Autodesk Inventor part; units mm, degrees
note: some values were not read from the file. Chosen so that the rebuilt part matches the saved one: direction of "Hole2".
(part 15 of 20)
  ellipse E161 centre (8.880264, -22.251224) end of major axis (8.019961, -22.341246) minor radius 0.036963 (9.7365, -22.165406) -> (8.039242, -22.346892) ccw
  ellipse E162 centre (8.776287, -21.257563) end of major axis (9.63659, -21.167541) minor radius 0.036963 (9.63659, -21.167541) -> (8.396683, -21.26386) ccw
  line L202 (9.63659, -21.167541) -> (9.740566, -22.161202)
  line L203 (7.930132, -21.482796) -> (8.019961, -22.341246)
  ellipse E163 centre (-8.87268, -22.249874) end of major axis (-9.732969, -22.159721) minor radius 0.036963 (-8.012398, -22.340088) -> (-9.728903, -22.163926) ccw
  ellipse E164 centre (-8.768552, -21.256229) end of major axis (-9.628841, -21.166076) minor radius 0.036963 (-8.388949, -21.262584) -> (-9.628841, -21.166076) ccw
  line L204 (-7.922432, -21.48159) -> (-8.01239, -22.340027)
  line L205 (-9.628841, -21.166076) -> (-9.732969, -22.159721)
  ellipse E165 centre (7.061717, -21.958191) end of major axis (7.924512, -21.896479) minor radius 0.002538 (7.708444, -21.913617) -> (6.964147, -21.962642) ccw
  line L206 (7.895215, -21.486873) -> (7.924512, -21.896479)
  ellipse E166 centre (9.777958, -21.218746) end of major axis (10.234812, -21.230292) minor radius 0.076505 (9.950925, -21.152163) -> (9.397885, -21.166946) ccw
  ellipse E167 centre (9.777958, -21.218746) end of major axis (10.642682, -21.2406) minor radius 0.144806 (10.484841, -21.319542) -> (9.2764, -21.088429) ccw
  ellipse E168 centre (9.802866, -20.233173) end of major axis (10.66759, -20.255027) minor radius 0.144806 (10.66759, -20.255027) -> (9.58532, -20.087637) ccw
  line L207 (10.66759, -20.255027) -> (10.642682, -21.2406)
  ellipse E169 centre (6.464823, -23.995199) end of major axis (6.018599, -24.093856) minor radius 0.001467 (6.792496, -23.921734) -> (6.030212, -24.091628) ccw
  ellipse E170 centre (6.464823, -23.995199) end of major axis (7.309427, -23.808464) minor radius 0.002777 (6.875465, -23.901925) -> (5.784426, -24.143943) ccw
  ellipse E171 centre (6.248946, -23.018784) end of major axis (7.093549, -22.832049) minor radius 0.002777 (6.975473, -22.856706) -> (5.668507, -23.145047) ccw
  line L208 (9.778285, -23.009543) -> (9.789898, -23.111986)
  line L209 (-9.770816, -23.008056) -> (-9.782444, -23.110498)
  ellipse E172 centre (-6.457505, -23.994216) end of major axis (-6.011296, -24.092941) minor radius 0.001467 (-6.022908, -24.090711) -> (-6.785166, -23.920701) ccw
  ellipse E173 centre (-6.457505, -23.994216) end of major axis (-5.61293, -24.18108) minor radius 0.002777 (-5.926087, -24.109581) -> (-6.868132, -23.90088) ccw
  ellipse E174 centre (-6.241479, -23.017834) end of major axis (-5.396904, -23.204697) minor radius 0.002777 (-5.843014, -23.103486) -> (-6.967981, -22.855645) ccw
  ellipse E175 centre (6.473855, -24.120964) end of major axis (6.919711, -24.020659) minor radius 0.077418 (6.673265, -24.148388) -> (6.070638, -24.174996) ccw
  ellipse E176 centre (6.473855, -24.120964) end of major axis (7.317762, -23.931109) minor radius 0.146534 (6.015845, -24.094803) -> (5.928892, -24.125217) ccw
  ellipse E177 centre (6.473855, -24.120964) end of major axis (7.317762, -23.931109) minor radius 0.146534 (6.927924, -24.148435) -> (7.27682, -23.899258) ccw
  line L210 (7.310373, -23.898267) -> (7.317762, -23.931109)
  ellipse E178 centre (-6.466555, -24.11998) end of major axis (-6.912396, -24.019607) minor radius 0.077418 (-6.057832, -24.177428) -> (-6.579408, -24.172057) ccw
  ellipse E179 centre (-6.466555, -24.11998) end of major axis (-5.622676, -24.309964) minor radius 0.146534 (-5.986709, -24.101247) -> (-6.008541, -24.093889) ccw
  ellipse E180 centre (-6.466555, -24.11998) end of major axis (-7.310434, -23.929997) minor radius 0.146534 (-7.269487, -23.898152) -> (-6.709989, -24.210547) ccw
  line L211 (-7.30304, -23.897155) -> (-7.310434, -23.929997)
  ellipse E181 centre (5.239934, -22.974099) end of major axis (6.04636, -22.661205) minor radius 0.002657 (5.413745, -22.903878) -> (5.065481, -23.039004) ccw
  ellipse E182 centre (4.878209, -22.04182) end of major axis (5.684634, -21.728925) minor radius 0.002657 (5.186609, -21.919528) -> (4.879859, -22.03833) ccw
  ellipse E183 centre (7.817682, -22.838707) end of major axis (8.648839, -22.599117) minor radius 0.158003 (7.952236, -22.639269) -> (7.749399, -22.694025) ccw
  ellipse E184 centre (7.817682, -22.838707) end of major axis (8.648839, -22.599117) minor radius 0.158003 (8.34332, -22.565329) -> (8.005856, -22.626461) ccw
  ellipse E185 centre (-9.875894, -23.012969) end of major axis (-10.332313, -23.03601) minor radius 0.081679 (-9.648403, -22.930955) -> (-9.779917, -23.088231) ccw
  ellipse E186 centre (-9.875894, -23.012969) end of major axis (-10.739794, -23.05658) minor radius 0.1546 (-9.405736, -22.860133) -> (-9.792131, -23.162938) ccw
  ellipse E187 centre (-9.925499, -22.030322) end of major axis (-10.789399, -22.073932) minor radius 0.1546 (-9.702595, -21.86988) -> (-10.789399, -22.073932) ccw
  line L212 (-10.789399, -22.073932) -> (-10.739794, -23.05658)
  ellipse E188 centre (-7.289451, -23.895158) end of major axis (-7.745819, -23.871138) minor radius 0.00147 (-6.894969, -23.916661) -> (-7.061668, -23.908422) ccw
  ellipse E189 centre (-7.289451, -23.895158) end of major axis (-8.153255, -23.849694) minor radius 0.002783 (-6.785011, -23.919446) -> (-7.303056, -23.897228) ccw
  ellipse E190 centre (-7.236891, -22.896545) end of major axis (-6.373087, -22.94201) minor radius 0.002783 (-6.4941, -22.934218) -> (-6.64737, -22.925537) ccw
  ellipse E191 centre (-7.236891, -22.896545) end of major axis (-8.100696, -22.851081) minor radius 0.002783 (-6.734833, -22.920702) -> (-8.100696, -22.851081) ccw
  line L213 (-8.100696, -22.851081) -> (-8.153255, -23.849694)
  ellipse E192 centre (6.236662, -22.702312) end of major axis (5.390447, -22.881603) minor radius 0.130549 (5.390447, -22.881603) -> (7.082877, -22.523021) ccw
  ellipse E193 centre (6.031764, -21.735234) end of major axis (5.185549, -21.914525) minor radius 0.130549 (5.297902, -21.82051) -> (6.83605, -21.610541) ccw
  line L214 (6.888255, -21.604445) -> (7.082877, -22.523021)
  line L215 (5.185549, -21.914525) -> (5.390447, -22.881603)
  ellipse E194 centre (9.046219, -24.203626) end of major axis (9.500344, -24.152445) minor radius 0.009734
  ellipse E195 centre (9.046219, -24.203626) end of major axis (8.18666, -24.300499) minor radius 0.018424 (8.42964, -24.286001) -> (8.202222, -24.302214) ccw
  ellipse E196 centre (8.934252, -23.210142) end of major axis (8.074693, -23.307015) minor radius 0.018424 (9.79381, -23.113269) -> (8.131366, -23.293966) ccw
  line L216 (9.79381, -23.113269) -> (9.905777, -24.106752)
  line L217 (8.136212, -23.852872) -> (8.18666, -24.300499)
  ellipse E197 centre (-9.038932, -24.20225) end of major axis (-9.493049, -24.151001) minor radius 0.009734
  ellipse E198 centre (-9.038932, -24.20225) end of major axis (-9.898475, -24.105246) minor radius 0.018424 (-8.182768, -24.297185) -> (-8.449093, -24.282273) ccw
  ellipse E199 centre (-8.926814, -23.208784) end of major axis (-9.786357, -23.11178) minor radius 0.018424 (-8.123941, -23.29273) -> (-9.786357, -23.11178) ccw
  line L218 (-9.786357, -23.11178) -> (-9.898475, -24.105246)
  ellipse E200 centre (-6.229147, -22.701364) end of major axis (-7.075334, -22.521944) minor radius 0.130549 (-7.075334, -22.521944) -> (-5.382959, -22.880783) ccw
  ellipse E201 centre (-6.024101, -21.734318) end of major axis (-6.870289, -21.554898) minor radius 0.130549 (-6.828368, -21.609501) -> (-5.209084, -21.866915) ccw
  line L219 (-5.177914, -21.913737) -> (-5.382959, -22.880783)
  line L220 (-6.880573, -21.603398) -> (-7.075334, -22.521944)
  ellipse E202 centre (7.296785, -23.896267) end of major axis (6.840413, -23.920218) minor radius 0.00147 (7.068999, -23.909497) -> (6.9023, -23.91771) ccw
  ellipse E203 centre (7.296785, -23.896267) end of major axis (8.160596, -23.850934) minor radius 0.002783 (7.31039, -23.898339) -> (6.792341, -23.920478) ccw
  ellipse E204 centre (7.244377, -22.897647) end of major axis (8.108188, -22.852314) minor radius 0.002783 (6.654851, -22.926548) -> (6.50158, -22.935206) ccw
  ellipse E205 centre (7.244377, -22.897647) end of major axis (8.108188, -22.852314) minor radius 0.002783 (8.108188, -22.852314) -> (6.742315, -22.921727) ccw
  line L221 (8.108188, -22.852314) -> (8.160596, -23.850934)
  ellipse E206 centre (9.883362, -23.014472) end of major axis (10.339777, -23.037582) minor radius 0.081679 (9.787373, -23.089719) -> (9.655883, -22.932423) ccw
  ellipse E207 centre (9.883362, -23.014472) end of major axis (10.747255, -23.058214) minor radius 0.1546 (9.799576, -23.164428) -> (9.413227, -22.861565) ccw
  ellipse E208 centre (9.933116, -22.031832) end of major axis (10.797009, -22.075574) minor radius 0.1546 (10.797009, -22.075574) -> (9.710237, -21.871357) ccw
  line L222 (10.797009, -22.075574) -> (10.747255, -23.058214)
  ellipse E209 centre (-7.810188, -22.837519) end of major axis (-6.979067, -23.077235) minor radius 0.158003 (-7.741883, -22.692847) -> (-7.816372, -22.671587) ccw
  ellipse E210 centre (-5.23246, -22.973303) end of major axis (-4.426082, -23.28632) minor radius 0.002657 (-5.102543, -23.020921) -> (-5.235934, -22.969105) ccw
  ellipse E211 centre (-4.870593, -22.041078) end of major axis (-4.064215, -22.354095) minor radius 0.002657 (-4.916775, -22.020307) -> (-5.105229, -21.947273) ccw
  ellipse E212 centre (8.55857, -18.364881) end of major axis (9.419561, -18.281692) minor radius 0.221488 (9.139361, -18.148216) -> (9.043274, -18.137267) ccw
  ellipse E213 centre (-8.550395, -18.36358) end of major axis (-7.689418, -18.4469) minor radius 0.221488 (-9.035064, -18.135893) -> (-9.131153, -18.146827) ccw
  ellipse E214 centre (-9.638197, -19.369972) end of major axis (-9.181207, -19.366996) minor radius 0.071862 (-9.5006, -19.300569) -> (-9.830873, -19.306032) ccw
  ellipse E215 centre (-9.638197, -19.369972) end of major axis (-10.503179, -19.375606) minor radius 0.13602 (-9.494183, -19.234934) -> (-10.501861, -19.36795) ccw
  ellipse E216 centre (-9.644629, -18.382434) end of major axis (-10.509611, -18.388068) minor radius 0.13602 (-9.049152, -18.279994) -> (-10.504657, -18.37336) ccw
  ellipse E217 centre (8.735192, -20.282112) end of major axis (9.19003, -20.237714) minor radius 0.026267 (9.1877, -20.24076) -> (9.187114, -20.235158) ccw
  ellipse E218 centre (8.735192, -20.282112) end of major axis (9.5961, -20.198076) minor radius 0.049718 (9.586329, -20.206816) -> (8.550212, -20.251321) ccw
  ellipse E219 centre (8.638201, -19.288488) end of major axis (9.499109, -19.204451) minor radius 0.049718 (9.499109, -19.204451) -> (8.704737, -19.23221) ccw
  line L223 (9.499109, -19.204451) -> (9.5961, -20.198076)
  ellipse E220 centre (-8.727309, -20.280784) end of major axis (-9.18214, -20.236316) minor radius 0.026267 (-9.179223, -20.233761) -> (-9.17981, -20.239364) ccw
  ellipse E221 centre (-8.727309, -20.280784) end of major axis (-9.588204, -20.196617) minor radius 0.049718 (-8.542324, -20.250021) -> (-9.578434, -20.205359) ccw
  ellipse E222 centre (-8.630166, -19.287175) end of major axis (-9.491062, -19.203007) minor radius 0.049718 (-8.696694, -19.230887) -> (-9.491062, -19.203007) ccw
  line L224 (-9.491062, -19.203007) -> (-9.588204, -20.196617)
  ellipse E223 centre (9.646219, -19.371439) end of major axis (10.103209, -19.374485) minor radius 0.071862 (9.838905, -19.307528) -> (9.508633, -19.302015) ccw
  ellipse E224 centre (9.646219, -19.371439) end of major axis (10.5112, -19.377204) minor radius 0.13602 (10.509883, -19.369548) -> (9.502226, -19.236378) ccw
  ellipse E225 centre (9.652802, -18.383902) end of major axis (10.517782, -18.389667) minor radius 0.13602 (10.512831, -18.374958) -> (9.05734, -18.281371) ccw
  ellipse E226 centre (0.009553, 53.506137) end of major axis (0.075525, 54.246444) minor radius 0.194882 (0.21457, 53.727796) -> (-0.195464, 53.284479) ccw
  line L225 (-0.195616, 51.274821) -> (-0.195464, 53.284479)
  line L226 (0.214417, 51.717553) -> (0.21457, 53.727796)
  ellipse E227 centre (2.143874, 53.506396) end of major axis (2.287088, 54.260493) minor radius 0.195462 (2.370981, 53.706836) -> (2.096124, 54.036091) ccw
  line L227 (-0.341173, 31.740705) -> (-0.256979, 32.544836)
  line L228 (2.209519, 52.164737) -> (2.370981, 53.706836)
  ellipse E228 centre (-2.124767, 53.50672) end of major axis (-2.140806, 54.274124) minor radius 0.195482 (-2.098936, 54.257488) -> (-2.305492, 53.26384) ccw
  line L229 (-2.200438, 52.259018) -> (-2.305492, 53.26384)
  line L230 (0.356969, 31.740652) -> (0.272897, 32.544796)
  ellipse E229 centre (0.0094, 51.496187) end of major axis (0.075622, 52.233172) minor radius 0.194809 (0.214417, 51.717553) -> (-0.195616, 51.274821) ccw
  line L231 (-0.196874, 34.739571) -> (-0.195616, 51.274821)
  line L232 (0.213126, 34.73954) -> (0.214417, 51.717553)
  ellipse E230 centre (2.174873, 51.495886) end of major axis (2.327161, 52.248199) minor radius 0.195466 (2.404376, 51.693529) -> (2.105864, 51.960619) ccw
  line L233 (-1.161209, 24.726698) -> (-0.341156, 31.740871)
  line L234 (0.224889, 33.051688) -> (2.404376, 51.693529)
  line L235 (-0.197636, 24.724772) -> (-0.197141, 31.229224)
  line L236 (0.212364, 24.724741) -> (0.212859, 31.229193)
  ellipse E231 centre (-2.156072, 51.496216) end of major axis (-2.181353, 52.263368) minor radius 0.195478 (-2.116003, 52.223205) -> (-2.333848, 51.251129) ccw
  line L237 (-0.208894, 33.051721) -> (-2.333848, 51.251129)
  line L238 (1.175938, 24.72652) -> (0.356952, 31.740818)
  ellipse E232 centre (0.009707, 55.534244) end of major axis (0.073644, 56.299137) minor radius 0.195472 (0.214724, 55.757114) -> (-0.195309, 55.311374) ccw
  line L239 (-0.195311, 55.290346) -> (-0.195309, 55.311374)
  line L240 (0.214723, 55.734095) -> (0.214724, 55.757114)
  ellipse E233 centre (0.009706, 55.51222) end of major axis (0.075476, 56.255172) minor radius 0.19494 (0.214723, 55.734095) -> (-0.195311, 55.290346) ccw
  line L241 (-0.195464, 53.284479) -> (-0.195311, 55.290346)
  line L242 (0.21457, 53.727796) -> (0.214723, 55.734095)
  ellipse E234 centre (2.127756, 55.512884) end of major axis (2.2636, 56.268331) minor radius 0.195467 (2.352894, 55.715465) -> (1.902618, 55.310302) ccw
  ellipse E235 centre (-0.793704, 24.716213) end of major axis (-0.58962, 24.696853) minor radius 0.000002 (-0.58962, 24.696853) -> (-0.835491, 24.720179) ccw
  line L243 (-0.257064, 32.543938) -> (-0.208885, 33.051813)
  line L244 (0.213336, 37.502674) -> (1.902618, 55.310302)
  line L245 (-0.58962, 24.696853) -> (-0.197323, 28.832262)
  line L246 (2.211634, 54.22637) -> (2.352894, 55.715465)
  ellipse E236 centre (-2.108345, 55.513206) end of major axis (-2.116886, 56.280719) minor radius 0.195476 (-1.925268, 55.754376) -> (-2.291421, 55.272036) ccw
  ellipse E237 centre (0.808431, 24.716091) end of major axis (0.604345, 24.696762) minor radius 0.000002 (0.850219, 24.720051) -> (0.604345, 24.696762) ccw
  line L247 (0.604345, 24.696762) -> (0.212677, 28.832231)
  line L248 (-2.193994, 54.243342) -> (-2.291421, 55.272036)
  line L249 (0.272982, 32.543898) -> (0.224881, 33.05178)
  line L250 (-0.196664, 37.502705) -> (-1.925268, 55.754376)
  line L251 (-9.047868, -18.018858) -> (-9.022159, -18.0039)
  line L252 (-9.106303, -17.898872) -> (-9.099175, -17.900444)
  line L253 (-9.132668, -17.914212) -> (-9.106303, -17.898872)
  line L254 (-9.106303, -17.898872) -> (-9.103206, -17.868962)
  line L255 (-10.711204, -17.866226) -> (-10.693895, -17.867036)
  line L256 (-10.693895, -17.867036) -> (-10.646494, -17.847198)
  line L257 (-10.542988, -17.803879) -> (-10.509871, -17.790019)
  line L258 (-10.338718, -17.71839) -> (-10.314571, -17.708284)
  line L259 (-10.507779, -17.699245) -> (-10.314571, -17.708284)
  line L260 (-10.589465, -17.733432) -> (-10.507779, -17.699245)
  line L261 (-10.314571, -17.708284) -> (-10.314603, -17.707039)
  line L262 (-10.507779, -17.699245) -> (-10.509198, -17.642731)
  line L263 (-10.555517, -15.798913) -> (-10.555525, -15.79856)
  line L264 (-10.608119, -13.704923) -> (-10.608743, -13.680109)
  line L265 (-9.94401, -17.647378) -> (-9.981118, -17.662908)
  line L266 (-9.944338, -17.634328) -> (-9.94401, -17.647378)
  line L267 (-9.94401, -17.647378) -> (-9.82656, -17.652873)
  line L268 (-9.676661, -17.659886) -> (-9.19249, -17.682536)
  line L269 (9.239478, -17.73124) -> (9.266389, -17.728982)
  line L270 (9.509904, -17.708556) -> (9.518634, -17.707823)
  line L271 (9.773763, -17.64453) -> (9.799149, -17.651722)
  line L272 (9.714512, -17.6495) -> (9.773763, -17.64453)
  line L273 (9.773763, -17.64453) -> (9.774235, -17.625861)
  line L274 (10.194358, -17.601742) -> (10.191995, -17.695228)
  line L275 (10.368223, -17.680446) -> (10.191995, -17.695228)
  line L276 (10.469835, -13.659859) -> (10.469373, -13.678124)
  line L277 (10.416258, -15.779768) -> (10.415723, -15.800971)
  line L278 (10.369921, -17.613254) -> (10.368223, -17.680446)
  line L279 (10.191995, -17.695228) -> (10.315866, -17.730322)
  line L280 (10.598304, -17.810338) -> (10.611283, -17.814015)
  line L281 (10.368223, -17.680446) -> (10.526706, -17.725345)
  line L282 (10.67671, -17.900341) -> (10.658231, -17.895106)
  line L283 (9.134915, -17.754095) -> (9.147769, -17.756408)
  line L284 (-10.64598, -17.972818) -> (-10.871518, -17.96517)
  line L285 (-10.959481, -18.003583) -> (-10.871518, -17.96517)
  line L286 (-10.643886, -18.014285) -> (-10.959481, -18.003583)
  line L287 (-10.959481, -18.003583) -> (-10.961848, -17.956702)
  line L288 (-11.169241, -17.911708) -> (-10.978836, -17.918164)
  line L289 (-11.172014, -17.856777) -> (-11.169241, -17.911708)
  line L290 (-10.978836, -17.918164) -> (-10.572528, -17.740733)
  line L291 (-10.762932, -17.734276) -> (-10.572528, -17.740733)
  line L292 (-11.169241, -17.911708) -> (-10.762932, -17.734276)
  line L293 (-10.572528, -17.740733) -> (-10.572852, -17.734313)
  line L294 (-10.762932, -17.734276) -> (-10.763409, -17.724824)
  line L295 (-10.395036, -13.665397) -> (-10.393502, -13.695801)
  line L296 (9.924361, -17.718581) -> (9.927437, -17.718404)
  line L297 (10.142861, -17.706037) -> (10.201617, -17.702664)
  line L298 (10.094508, -17.665104) -> (10.201617, -17.702664)
  line L299 (10.038776, -17.668304) -> (10.094508, -17.665104)
  line L300 (10.201617, -17.702664) -> (10.201852, -17.698021)
  line L301 (10.094508, -17.665104) -> (10.097435, -17.607306)
  line L302 (10.189858, -15.781958) -> (10.190459, -15.770084)
  line L303 (10.502946, -17.727127) -> (10.502742, -17.731166)
  line L304 (10.683071, -17.720814) -> (10.502742, -17.731166)
  line L305 (10.684038, -17.701713) -> (10.683071, -17.720814)
  line L306 (10.502742, -17.731166) -> (10.99748, -17.904656)
  line L307 (11.17781, -17.894303) -> (10.99748, -17.904656)
  line L308 (10.683071, -17.720814) -> (11.17781, -17.894303)
  line L309 (11.17781, -17.894303) -> (11.180482, -17.841516)
  line L310 (11.027881, -17.992409) -> (10.920773, -17.954849)
  line L311 (11.03036, -17.943446) -> (11.027881, -17.992409)
  line L312 (10.920773, -17.954849) -> (10.654432, -17.97014)
  line L313 (11.027881, -17.992409) -> (10.652212, -18.013976)
  line L314 (-10.130994, -17.702463) -> (-10.064078, -17.680853)
  line L315 (-10.25215, -17.667357) -> (-10.064078, -17.680853)
  line L316 (-10.359884, -17.702149) -> (-10.25215, -17.667357)
  line L317 (-10.064078, -17.680853) -> (-10.064408, -17.630256)
  line L318 (-10.076474, -15.77766) -> (-10.079226, -15.355191)
  line L319 (-10.25215, -17.667357) -> (-10.252433, -17.623881)
  line L320 (-10.264515, -15.768863) -> (-10.264554, -15.76289)
  line L321 (-10.278215, -13.665506) -> (-10.278389, -13.638755)
  line L322 (9.002945, -17.724125) -> (9.727913, -17.663671)
  line L323 (9.623702, -17.634324) -> (9.727913, -17.663671)
  line L324 (9.34766, -17.657343) -> (9.623702, -17.634324)
  line L325 (9.727913, -17.663671) -> (9.727979, -17.653778)
  line L326 (9.623702, -17.634324) -> (9.62385, -17.612121)
  line L327 (9.650348, -13.636669) -> (9.650555, -13.605672)
  line L328 (-7.427478, 0.491287) -> (-8.422703, 0.595367)
  line L329 (-11.2211, 1.390746) -> (-8.370636, 1.092648)
  ellipse E238 centre (-9.068011, 1.165222) end of major axis (-11.554419, 1.425556) minor radius 0.000177 (-11.2211, 1.390746) -> (-11.554419, 1.425556) ccw
  line L330 (-11.752095, -0.462417) -> (-11.554419, 1.425556)
  line L331 (8.433761, 0.594085) -> (7.43852, 0.490157)
  line L332 (8.38177, 1.091374) -> (11.23228, 1.389038)
  ellipse E239 centre (9.079156, 1.163842) end of major axis (11.565604, 1.423798) minor radius 0.000177 (11.565604, 1.423798) -> (11.23228, 1.389038) ccw
  line L333 (11.565604, 1.423798) -> (11.762993, -0.464205)
  ellipse E240 centre (-8.794361, -3.325086) end of major axis (-9.04267, -3.296056) minor radius 0.000013
  ellipse E241 centre (-7.725925, -3.450033) end of major axis (-8.318787, -3.380719) minor radius 0.00003 (-8.267942, -3.386651) -> (-8.267945, -3.386675) ccw
  ellipse E242 centre (-11.214903, -3.042309) end of major axis (-10.424441, -3.134724) minor radius 0.000039 (-11.564379, -3.001416) -> (-11.564487, -3.001473) ccw
  line L334 (-8.26792, -3.386459) -> (-12.108041, -2.937836)
  ellipse E243 centre (-9.957751, -3.189298) end of major axis (-12.440838, -2.898991) minor radius 0.000126 (-12.100681, -2.938696) -> (-12.440795, -2.898995) ccw
  line L335 (-11.817734, -0.454749) -> (-8.971383, -0.787274)
  ellipse E244 centre (-9.667444, -0.706211) end of major axis (-12.150531, -0.415904) minor radius 0.000126 (-11.817734, -0.454749) -> (-12.150531, -0.415904) ccw
  line L336 (-12.440838, -2.898991) -> (-12.150531, -0.415904)
  ellipse E245 centre (-4.295954, -3.851144) end of major axis (-12.73845, -2.864101) minor radius 0.000429 (-12.316833, -2.913529) -> (-11.564641, -3.001555) ccw
  line L337 (-8.035802, -1.399974) -> (-9.029444, -1.283892)
  ellipse E246 centre (8.804824, -3.326425) end of major axis (8.55651, -3.355418) minor radius 0.000013
  ellipse E247 centre (7.736368, -3.451209) end of major axis (8.329241, -3.381985) minor radius 0.00003 (8.278398, -3.387934) -> (8.278395, -3.387909) ccw
  ellipse E248 centre (4.306337, -3.851799) end of major axis (12.748983, -2.866039) minor radius 0.000429 (11.575153, -3.003315) -> (12.327357, -2.915403) ccw
  ellipse E249 centre (9.968234, -3.190813) end of major axis (12.451365, -2.900884) minor radius 0.000126 (12.327357, -2.915403) -> (12.118562, -2.939678) ccw
  line L338 (12.118562, -2.939678) -> (8.278373, -3.387717)
  line L339 (8.982231, -0.78864) -> (11.828633, -0.456547)
  ellipse E250 centre (9.678304, -0.707682) end of major axis (12.161436, -0.417753) minor radius 0.000126 (12.161436, -0.417753) -> (11.828633, -0.456547) ccw
  line L340 (12.161436, -0.417753) -> (12.451365, -2.900884)
  ellipse E251 centre (11.225408, -3.044015) end of major axis (10.434932, -3.13631) minor radius 0.000039 (11.574998, -3.003233) -> (11.574891, -3.003175) ccw
  line L341 (9.040217, -1.285266) -> (8.046557, -1.401197)
  line L342 (-6.927395, 2.406749) -> (-7.923221, 2.501197)
  line L343 (-10.728785, 3.269529) -> (-7.876002, 2.998962)
  ellipse E252 centre (-8.573487, 3.065058) end of major axis (-11.062314, 3.301155) minor radius 0.000028 (-10.728785, 3.269529) -> (-11.062314, 3.301155) ccw
  line L344 (-11.24332, 1.39307) -> (-11.062314, 3.301155)
  line L345 (4.093757, 2.586746) -> (4.005682, 2.601143)
  line L346 (-3.994318, 2.601751) -> (-4.082396, 2.587368)
  line L347 (-5.778862, 2.808104) -> (-4.994293, 2.936222)
  line L348 (5.005707, 2.935462) -> (5.790257, 2.807224)
  line L349 (7.93457, 2.499991) -> (6.938729, 2.405694)
  line L350 (7.887426, 2.997763) -> (10.74025, 3.267897)
  ellipse E253 centre (8.584922, 3.063753) end of major axis (11.073784, 3.299472) minor radius 0.000028 (11.073784, 3.299472) -> (10.74028, 3.267899) ccw
  line L351 (11.073784, 3.299472) -> (11.2545, 1.391359)
  spline S0 degree 3 poles (-6.270261, 3.386408) (-6.22537, 3.406214) (-6.136517, 3.445415) (-6.003702, 3.501576) (-5.872921, 3.555061) (-5.702594, 3.621964) (-5.493969, 3.699586) (-5.32639, 3.754652) (-5.244083, 3.781698) knots 0 0 0 0 0.13378969 0.26480564 0.39318317 0.51905417 0.76378306 1 1 1 1
  line L352 (-6.325383, 2.859948) -> (-6.270261, 3.386408)
  spline S1 degree 3 poles (-7.39801, 3.74416) (-7.41143, 3.74308) (-7.437886, 3.74095) (-7.477008, 3.738874) (-7.514824, 3.737738) (-7.551134, 3.737655) (-7.585748, 3.738663) (-7.618528, 3.740793) (-7.649392, 3.743982) (-7.678296, 3.74818) (-7.705199, 3.753335) (-7.730058, 3.759394) (-7.752833, 3.766308) (-7.773504, 3.774031) (-7.792228, 3.782612) (-7.809155, 3.79217) (-7.824593, 3.802616) (-7.833739, 3.810627) (-7.838227, 3.814557) knots 0 0 0 0 0.08847523 0.17442408 0.25743028 0.33708941 0.41301484 0.48496567 0.5529194 0.61687848 0.67685349 0.73286663 0.78495643 0.83318442 0.87777974 0.92016243 0.96082909 1 1 1 1
  ellipse E254 centre (-3.138193, 3.058154) end of major axis (-8.569503, 3.626827) minor radius 0.000387 (-6.270263, 3.386408) -> (-8.569503, 3.626827) ccw
  line L353 (-8.255694, 3.881151) -> (-8.569503, 3.626827)
  line L354 (-8.627777, 3.070263) -> (-8.569503, 3.626827)
  spline S2 degree 3 poles (-3.144169, 3.522717) (-3.101581, 3.546955) (-3.017287, 3.594929) (-2.891037, 3.664227) (-2.766531, 3.730668) (-2.604086, 3.814476) (-2.404663, 3.912851) (-2.243738, 3.984658) (-2.164694, 4.019928) knots 0 0 0 0 0.13376268 0.26475964 0.39312605 0.51899363 0.76373828 1 1 1 1
  line L355 (-3.144182, 3.340991) -> (-3.144169, 3.522717)
  line L356 (3.155673, 3.522238) -> (3.155659, 3.340512)
  spline S3 degree 3 poles (2.176274, 4.019598) (2.255312, 3.984316) (2.416226, 3.912485) (2.615634, 3.814079) (2.778066, 3.730246) (2.902563, 3.663786) (3.028802, 3.594469) (3.113089, 3.546482) (3.155673, 3.522238) knots 0 0 0 0 0.23626172 0.48100637 0.60687395 0.73524036 0.86623732 1 1 1 1
  line L357 (-2.164694, 4.019928) -> (2.176274, 4.019598)
  ellipse E255 centre (0.005755, 3.555498) end of major axis (-4.955245, 3.555876) minor radius 0.5163 (2.68037, 3.990137) -> (2.176274, 4.019598) ccw
  ellipse E256 centre (0.005755, 3.555498) end of major axis (-4.955245, 3.555876) minor radius 0.5163 (-2.164694, 4.019928) -> (-2.668795, 3.990544) ccw
  ellipse E257 centre (0.005717, 3.058213) end of major axis (5.466717, 3.057798) minor radius 0.568336 (5.303063, 3.195907) -> (3.155673, 3.522238) ccw
  ellipse E258 centre (0.005717, 3.058213) end of major axis (-5.455283, 3.058629) minor radius 0.568336 (-3.144169, 3.522717) -> (-5.291609, 3.196713) ccw
  line L358 (6.281745, 3.385454) -> (6.336786, 2.858985)
  spline S4 degree 3 poles (5.255626, 3.780899) (5.337929, 3.753841) (5.5055, 3.698749) (5.714113, 3.621096) (5.884429, 3.554167) (6.015203, 3.500662) (6.148009, 3.44448) (6.236856, 3.405266) (6.281745, 3.385454) knots 0 0 0 0 0.23621694 0.48094583 0.60681683 0.73519436 0.86621031 1 1 1 1
  spline S5 degree 3 poles (7.849327, 3.813558) (7.844658, 3.809554) (7.835089, 3.801347) (7.818862, 3.790633) (7.800944, 3.780749) (7.781217, 3.771856) (7.759735, 3.763923) (7.736504, 3.756977) (7.711541, 3.751027) (7.684861, 3.746091) (7.656461, 3.74218) (7.626293, 3.739311) (7.594323, 3.737468) (7.56055, 3.736632) (7.525029, 3.736795) (7.487824, 3.737963) (7.448989, 3.740063) (7.422599, 3.742214) (7.409134, 3.743311) knots 0 0 0 0 0.04039145 0.08278851 0.12750015 0.17478558 0.22486002 0.27790108 0.33405492 0.39344169 0.45616024 0.52241148 0.59256068 0.66658365 0.74441779 0.82598879 0.91121312 1 1 1 1
  ellipse E259 centre (3.149626, 3.057676) end of major axis (8.581023, 3.625523) minor radius 0.000387 (8.581023, 3.625523) -> (6.281745, 3.385454) ccw
  line L359 (8.267252, 3.879894) -> (8.581023, 3.625523)
  line L360 (8.639212, 3.06895) -> (8.581023, 3.625523)
  spline S6 degree 3 poles (-5.798085, 5.31307) (-5.753389, 5.333312) (-5.664922, 5.373376) (-5.532661, 5.430829) (-5.402406, 5.485586) (-5.23274, 5.554145) (-5.024881, 5.633795) (-4.857846, 5.690492) (-4.775807, 5.718338) knots 0 0 0 0 0.13378969 0.26480564 0.39318317 0.51905417 0.76378306 1 1 1 1
  line L361 (-5.968571, 3.515891) -> (-5.798085, 5.31307)
  line L362 (-4.775807, 5.718338) -> (-3.980079, 5.642853)
  ellipse E260 centre (-2.615343, 5.51334) end of major axis (-7.554171, 5.981852) minor radius 0.000055 (-7.384376, 5.965759) -> (-7.554171, 5.981852) ccw
  ellipse E261 centre (-2.615343, 5.51334) end of major axis (-7.554171, 5.981852) minor radius 0.000055 (-4.775806, 5.718338) -> (-6.11123, 5.845009) ccw
  spline S7 degree 3 poles (-6.11123, 5.845009) (-6.1628, 5.829169) (-6.263815, 5.798141) (-6.413188, 5.757283) (-6.556182, 5.722285) (-6.691956, 5.693824) (-6.820794, 5.671951) (-6.942412, 5.657483) (-7.038947, 5.651776) (-7.110576, 5.652136) (-7.158813, 5.654891) (-7.202884, 5.659959) (-7.242634, 5.667172) (-7.277945, 5.676377) (-7.317413, 5.690502) (-7.358752, 5.713338) (-7.395931, 5.751237) (-7.416895, 5.798571) (-7.419451, 5.852124) (-7.408266, 5.909059) (-7.39259, 5.946264) (-7.384375, 5.965759) knots 0 0 0 0 0.10413454 0.20397599 0.29888876 0.38827472 0.47171081 0.55106733 0.62459732 0.65820388 0.68929134 0.71781594 0.74378428 0.76721832 0.78816557 0.82463321 0.85738378 0.88888098 0.92222056 0.95924484 1 1 1 1
  ellipse E262 centre (-2.662562, 5.015575) end of major axis (-8.099155, 5.531306) minor radius 0.000061 (-5.798127, 5.313074) -> (-8.099155, 5.531306) ccw
  line L363 (-7.554171, 5.981852) -> (-8.099155, 5.531306)
  ellipse E263 centre (-6.053301, 5.839497) end of major axis (-4.548756, 5.696772) minor radius 0.000017 (-7.384833, 5.965802) -> (-6.193955, 5.852823) ccw
  line L364 (-8.255694, 3.881151) -> (-8.099155, 5.531306)
  spline S8 degree 3 poles (-3.144023, 5.436372) (-3.101436, 5.460633) (-3.017142, 5.508654) (-2.890892, 5.578019) (-2.766386, 5.644525) (-2.603942, 5.728415) (-2.40452, 5.826886) (-2.243592, 5.898764) (-2.164548, 5.934068) knots 0 0 0 0 0.13376751 0.26476787 0.39313627 0.51900446 0.76374629 1 1 1 1
  line L365 (-3.144153, 3.722274) -> (-3.144023, 5.436372)
  line L366 (3.155818, 5.435893) -> (3.155688, 3.721795)
  spline S9 degree 3 poles (2.176419, 5.933738) (2.255458, 5.898422) (2.416375, 5.826519) (2.615781, 5.728018) (2.778213, 5.644104) (2.902709, 5.577579) (3.028948, 5.508194) (3.113234, 5.460161) (3.155818, 5.435893) knots 0 0 0 0 0.23625371 0.48099554 0.60686373 0.73523213 0.86623249 1 1 1 1
  line L367 (-2.164548, 5.934068) -> (2.176419, 5.933738)
  ellipse E264 centre (0.005903, 5.51312) end of major axis (-4.955097, 5.513497) minor radius 0.467946 (3.517763, 5.843374) -> (2.176419, 5.933738) ccw
  ellipse E265 centre (0.005903, 5.51312) end of major axis (-4.955097, 5.513497) minor radius 0.467946 (-2.164548, 5.934068) -> (-3.505905, 5.843909) ccw
  spline S10 degree 3 poles (-3.505905, 5.843909) (-3.546001, 5.825724) (-3.624987, 5.789901) (-3.742365, 5.739024) (-3.856274, 5.691531) (-3.966272, 5.647799) (-4.071856, 5.608053) (-4.173258, 5.572263) (-4.270803, 5.540603) (-4.36402, 5.513367) (-4.451024, 5.491279) (-4.52969, 5.475375) (-4.598495, 5.46587) (-4.6566, 5.462381) (-4.704799, 5.464591) (-4.743498, 5.472994) (-4.774986, 5.48663) (-4.788533, 5.50222) (-4.794828, 5.509466) knots 0 0 0 0 0.09648314 0.19006443 0.28034292 0.36693478 0.44946267 0.527566 0.60257164 0.67417927 0.74035842 0.79922956 0.84998037 0.89243012 0.92670891 0.95522625 0.97919149 1 1 1 1
  spline S11 degree 3 poles (4.806622, 5.508742) (4.800475, 5.501672) (4.787179, 5.486381) (4.755992, 5.47292) (4.71732, 5.46454) (4.669747, 5.461938) (4.613774, 5.464811) (4.549186, 5.473396) (4.475995, 5.487815) (4.394285, 5.507881) (4.304539, 5.533444) (4.207483, 5.56428) (4.10385, 5.600168) (3.994383, 5.640858) (3.879986, 5.686116) (3.719838, 5.752496) (3.599248, 5.806728) (3.517763, 5.843374) knots 0 0 0 0 0.02031374 0.04393674 0.07255557 0.10706143 0.14790384 0.19530387 0.24973648 0.31134419 0.37967367 0.4542385 0.53453299 0.62003981 0.71019877 0.8041769 1 1 1 1
  ellipse E266 centre (0.005866, 5.015349) end of major axis (5.466866, 5.014934) minor radius 0.515109 (5.160923, 5.184952) -> (3.155818, 5.435893) ccw
  ellipse E267 centre (0.005866, 5.015349) end of major axis (-5.455134, 5.015764) minor radius 0.515109 (-3.144023, 5.436372) -> (-5.149166, 5.185736) ccw
  line L368 (5.809862, 5.312187) -> (5.980074, 3.514982)
  spline S12 degree 3 poles (4.787645, 5.717611) (4.86968, 5.689752) (5.036706, 5.63303) (5.244552, 5.553348) (5.414209, 5.484763) (5.544455, 5.429986) (5.676708, 5.372514) (5.765168, 5.332436) (5.809862, 5.312187) knots 0 0 0 0 0.23621694 0.48094583 0.60681683 0.73519436 0.86621031 1 1 1 1
  line L369 (3.991905, 5.642247) -> (4.787645, 5.717611)
  ellipse E268 centre (2.62715, 5.512942) end of major axis (-2.311749, 5.045182) minor radius 0.000055 (6.124544, 5.844217) -> (4.789499, 5.717786) ccw
  ellipse E269 centre (2.62715, 5.512942) end of major axis (7.566049, 5.980702) minor radius 0.000055 (7.566049, 5.980702) -> (7.39625, 5.964635) ccw
  spline S13 degree 3 poles (7.396251, 5.964635) (7.404697, 5.944626) (7.420555, 5.907059) (7.431456, 5.850043) (7.428597, 5.797517) (7.408214, 5.751067) (7.371237, 5.713459) (7.31973, 5.684824) (7.254378, 5.664659) (7.17509, 5.652911) (7.0818, 5.649844) (6.97487, 5.654917) (6.855252, 5.668021) (6.724353, 5.688988) (6.583672, 5.717635) (6.435042, 5.75368) (6.280338, 5.795798) (6.176048, 5.827818) (6.123088, 5.844079) knots 0 0 0 0 0.04184874 0.07857029 0.11114659 0.14190435 0.17426777 0.21118388 0.25459927 0.30565856 0.36551927 0.43456112 0.51220716 0.59775966 0.69045627 0.7893544 0.8930296 1 1 1 1
  ellipse E270 centre (2.674293, 5.015169) end of major axis (8.110965, 5.530073) minor radius 0.000061 (8.110965, 5.530073) -> (5.809862, 5.312187) ccw
  line L370 (7.566049, 5.980702) -> (8.110965, 5.530073)
  line L371 (8.267252, 3.879894) -> (8.110965, 5.530073)
  ellipse E271 centre (-2.825792, 6.041844) end of major axis (-6.719508, 6.449526) minor radius 0.000278 (-3.185488, 6.079783) -> (-4.449778, 6.212133) ccw
  ellipse E272 centre (-4.764705, 6.245066) end of major axis (-4.565792, 6.224239) minor radius 0.000014 (-4.65593, 6.233665) -> (-4.565792, 6.224239) ccw
  line L372 (-4.565728, 6.224261) -> (-4.565792, 6.224239)
  ellipse E273 centre (-4.366815, 6.203434) end of major axis (-4.565728, 6.224261) minor radius 0.000014 (-4.449778, 6.212133) -> (-4.565728, 6.224261) ccw
  ellipse E274 centre (-2.825792, 6.041844) end of major axis (-6.172498, 6.392253) minor radius 0.000239 (-4.65593, 6.233665) -> (-6.172498, 6.392253) ccw
  line L373 (-6.172498, 6.392253) -> (-6.228633, 5.856113)
  ellipse E275 centre (-1.180484, 21.755945) end of major axis (-3.428197, 21.991286) minor radius 0.00016 (-3.154048, 21.962659) -> (-3.428197, 21.991286) ccw
  line L374 (-3.428197, 21.991286) -> (-3.724709, 20.044201)
  line L375 (1.755935, 5.93377) -> (1.75597, 6.393157)
  ellipse E276 centre (1.55597, 6.393172) end of major axis (1.75597, 6.393157) minor radius 0.020814 (1.75597, 6.393157) -> (1.639417, 6.412082) ccw
  ellipse E277 centre (0.005944, 6.041923) end of major axis (-3.909056, 6.042221) minor radius 0.407441 (1.639417, 6.412082) -> (-1.627474, 6.41233) ccw
  ellipse E278 centre (1.955967, 6.352368) end of major axis (1.755967, 6.352383) minor radius 0.020814 (1.755967, 6.352383) -> (1.846569, 6.334952) ccw
  ellipse E279 centre (-1.944033, 6.352664) end of major axis (-1.744033, 6.352649) minor radius 0.020814 (-1.834637, 6.335232) -> (-1.744033, 6.352649) ccw
  ellipse E280 centre (-1.54403, 6.393408) end of major axis (-1.74403, 6.393423) minor radius 0.020814 (-1.627474, 6.41233) -> (-1.74403, 6.393423) ccw
  line L376 (-1.74403, 6.393423) -> (-1.744065, 5.934036)
  ellipse E281 centre (0.005944, 6.041923) end of major axis (3.370944, 6.041667) minor radius 0.350202 (3.333804, 6.093559) -> (1.846569, 6.334952) ccw
  ellipse E282 centre (0.005944, 6.041923) end of major axis (-3.359056, 6.042179) minor radius 0.350202 (-1.834637, 6.335232) -> (-3.321909, 6.094066) ccw
  ellipse E283 centre (0.007139, 21.756125) end of major axis (2.267139, 21.755953) minor radius 0.235202 (1.045232, 21.964969) -> (-1.030923, 21.965127) ccw
  ellipse E284 centre (4.378727, 6.202769) end of major axis (4.577643, 6.223565) minor radius 0.000014 (4.577643, 6.223565) -> (4.461691, 6.211456) ccw
  ellipse E285 centre (2.837679, 6.041413) end of major axis (-1.056098, 5.634323) minor radius 0.000278 (4.461703, 6.211457) -> (3.197395, 6.079299) ccw
  line L377 (4.577707, 6.223544) -> (4.577643, 6.223565)
  ellipse E286 centre (4.776623, 6.244341) end of major axis (4.577707, 6.223544) minor radius 0.000014 (4.577707, 6.223544) -> (4.667846, 6.232956) ccw
  ellipse E287 centre (2.837679, 6.041413) end of major axis (6.184438, 6.391313) minor radius 0.000239 (6.184438, 6.391313) -> (4.667844, 6.232956) ccw
  line L378 (6.184438, 6.391313) -> (6.240492, 5.855165)
  ellipse E288 centre (1.194761, 21.755764) end of major axis (3.44251, 21.990764) minor radius 0.00016 (3.44251, 21.990764) -> (3.168357, 21.962178) ccw
  line L379 (3.44251, 21.990764) -> (3.738726, 20.043633)
  ellipse E289 centre (-1.532232, 19.787845) end of major axis (-3.776943, 20.050283) minor radius 0.000114 (-3.018809, 19.961733) -> (-3.776943, 20.050283) ccw
  line L380 (-3.776943, 20.050283) -> (-5.70867, 8.31801)
  line L381 (-5.757556, 8.021102) -> (-6.028223, 6.377217)
  ellipse E290 centre (0.005796, 4.094926) end of major axis (-3.909204, 4.095224) minor radius 0.45382 (0.724196, 4.540986) -> (0.620356, 4.543073) ccw
  ellipse E291 centre (0.005796, 4.094926) end of major axis (-3.909204, 4.095224) minor radius 0.45382 (0.346502, 4.546999) -> (-0.389801, 4.546453) ccw
  ellipse E292 centre (0.005796, 4.094926) end of major axis (-3.909204, 4.095224) minor radius 0.45382 (-0.608696, 4.543167) -> (-0.712537, 4.541095) ccw
  ellipse E293 centre (0.006989, 19.788414) end of major axis (2.266989, 19.788242) minor radius 0.261975 (1.715963, 19.959712) -> (-1.701959, 19.959972) ccw
  ellipse E294 centre (1.54621, 19.787611) end of major axis (3.790961, 20.049707) minor radius 0.000114 (3.790961, 20.049707) -> (3.032813, 19.961272) ccw
  line L382 (3.790961, 20.049707) -> (5.720904, 8.317141)
  line L383 (5.769745, 8.020225) -> (6.040161, 6.376299)
  ellipse E295 centre (-0.793704, 24.716213) end of major axis (-0.58962, 24.696853) minor radius 0.000002 (-0.58962, 24.696853) -> (-0.835491, 24.720179) ccw
  ellipse E296 centre (-0.834875, 24.282207) end of major axis (-2.064355, 24.398839) minor radius 0.000014 (-1.178308, 24.314799) -> (-2.064355, 24.398839) ccw
  line L384 (-2.064355, 24.398839) -> (-2.11659, 23.848204)
  arc A0 (-1.161194, 24.7267) -> (-2.064355, 24.398839) centre (-0.974939, 22.805716) ccw
  arc A1 (-0.483797, 24.672169) -> (-0.58962, 24.696853) centre (-0.974939, 22.805716) ccw
  ellipse E297 centre (-2.379246, 8.002167) end of major axis (-6.276748, 8.371895) minor radius 0.000044 (-3.017299, 8.062738) -> (-4.005136, 8.156443) ccw
  ellipse E298 centre (-2.473685, 7.006636) end of major axis (-6.371187, 7.376365) minor radius 0.000044 (-2.724099, 7.030435) -> (-4.099575, 7.160913) ccw
  line L385 (-4.121183, 8.16745) -> (-4.121211, 8.167448)
  line L386 (-4.215621, 7.171919) -> (-4.21565, 7.171918)
  ellipse E299 centre (-2.379246, 8.002167) end of major axis (-5.729206, 8.319954) minor radius 0.000037 (-4.211421, 8.176004) -> (-5.729206, 8.319954) ccw
  ellipse E300 centre (-2.473685, 7.006636) end of major axis (-5.823645, 7.324423) minor radius 0.000037 (-4.305859, 7.180473) -> (-5.582381, 7.30155) ccw
  line L387 (-5.729206, 8.319954) -> (-5.757557, 8.021097)
  ellipse E301 centre (-0.887112, 23.731551) end of major axis (-3.137011, 23.944983) minor radius 0.000025 (-1.971995, 23.834489) -> (-3.137011, 23.944983) ccw
  line L388 (-3.137011, 23.944983) -> (-3.415272, 21.98995)
  ellipse E302 centre (0.007331, 24.28219) end of major axis (1.242331, 24.282096) minor radius 0.116491 (1.193002, 24.314695) -> (-1.178335, 24.314876) ccw
  arc A2 (-0.196793, 24.724862) -> (-0.974318, 24.467446) centre (0.007218, 22.805682) ccw
  arc A3 (0.989007, 24.467296) -> (0.211522, 24.724831) centre (0.007218, 22.805682) ccw
  ellipse E303 centre (1.556041, 7.324774) end of major axis (1.756041, 7.324759) minor radius 0.018865 (1.756041, 7.324759) -> (1.639488, 7.341912) ccw
  line L389 (1.756041, 7.324759) -> (1.756117, 8.3203)
  ellipse E304 centre (1.556117, 8.320315) end of major axis (1.756117, 8.3203) minor radius 0.018865 (1.756117, 8.3203) -> (1.639564, 8.337454) ccw
  ellipse E305 centre (0.006093, 8.001973) end of major axis (-3.908907, 8.002271) minor radius 0.369282 (1.639564, 8.337454) -> (-1.627327, 8.337702) ccw
  ellipse E306 centre (0.006017, 7.006432) end of major axis (-3.908983, 7.00673) minor radius 0.369282 (1.639488, 7.341912) -> (-1.627403, 7.342161) ccw
  ellipse E307 centre (1.956114, 8.28333) end of major axis (1.756114, 8.283345) minor radius 0.018865 (1.756114, 8.283345) -> (1.846716, 8.267545) ccw
  ellipse E308 centre (-1.943886, 8.283626) end of major axis (-1.743886, 8.283611) minor radius 0.018865 (-1.83449, 8.267825) -> (-1.743886, 8.283611) ccw
  ellipse E309 centre (-1.543883, 8.320551) end of major axis (-1.743883, 8.320566) minor radius 0.018865 (-1.627327, 8.337702) -> (-1.743883, 8.320566) ccw
  ellipse E310 centre (-1.543959, 7.32501) end of major axis (-1.743959, 7.325025) minor radius 0.018865 (-1.627403, 7.342161) -> (-1.743959, 7.325025) ccw
  line L390 (-1.743883, 8.320566) -> (-1.743959, 7.325025)
  ellipse E311 centre (1.956038, 7.287788) end of major axis (1.756038, 7.287804) minor radius 0.018865 (1.756038, 7.287804) -> (1.84664, 7.272004) ccw
  line L391 (1.756038, 7.287804) -> (1.756041, 7.324759)
  ellipse E312 centre (-1.943962, 7.288085) end of major axis (-1.743962, 7.28807) minor radius 0.018865 (-1.834566, 7.272284) -> (-1.743962, 7.28807) ccw
  line L392 (-1.743959, 7.325025) -> (-1.743962, 7.28807)
  ellipse E313 centre (0.006093, 8.001973) end of major axis (3.371093, 8.001717) minor radius 0.317404 (3.256674, 8.083794) -> (1.846716, 8.267545) ccw
  ellipse E314 centre (0.006093, 8.001973) end of major axis (-3.358907, 8.002229) minor radius 0.317404 (-1.83449, 8.267825) -> (-3.244476, 8.084288) ccw
  ellipse E315 centre (0.006017, 7.006432) end of major axis (-3.358983, 7.006688) minor radius 0.317404 (-3.263823, 7.081628) -> (-3.333244, 7.045866) ccw
  ellipse E316 centre (0.006017, 7.006432) end of major axis (3.371017, 7.006176) minor radius 0.317404 (-1.834566, 7.272284) -> (-3.05482, 7.138532) ccw
  ellipse E317 centre (0.006017, 7.006432) end of major axis (3.371017, 7.006176) minor radius 0.317404 (3.066874, 7.138067) -> (1.84664, 7.272004) ccw
  ellipse E318 centre (0.006017, 7.006432) end of major axis (3.371017, 7.006176) minor radius 0.317404 (3.345284, 7.045359) -> (3.275869, 7.08113) ccw
  ellipse E319 centre (0.007289, 23.731528) end of major axis (2.267289, 23.731356) minor radius 0.213175 (1.986914, 23.834219) -> (-1.97232, 23.83452) ccw
  ellipse E320 centre (0.808431, 24.716091) end of major axis (0.604345, 24.696762) minor radius 0.000002 (0.850219, 24.720051) -> (0.604345, 24.696762) ccw
  ellipse E321 centre (0.849536, 24.282079) end of major axis (2.079034, 24.398524) minor radius 0.000014 (2.079034, 24.398524) -> (1.192974, 24.314619) ccw
  line L393 (2.079034, 24.398524) -> (2.131185, 23.847881)
  arc A4 (0.604345, 24.696762) -> (0.498518, 24.672095) centre (0.989376, 22.805566) ccw
  arc A5 (2.079034, 24.398524) -> (1.175924, 24.726522) centre (0.989376, 22.805566) ccw
  ellipse E322 centre (2.391431, 8.001804) end of major axis (-1.506128, 7.632669) minor radius 0.000044 (4.01786, 8.155882) -> (3.030053, 8.062331) ccw
  ellipse E323 centre (2.485719, 7.006259) end of major axis (-1.41184, 6.637124) minor radius 0.000044 (4.112146, 7.160337) -> (2.736701, 7.030073) ccw
  line L394 (4.133421, 8.16682) -> (4.133393, 8.166822)
  line L395 (4.227709, 7.171275) -> (4.22768, 7.171277)
  ellipse E324 centre (2.391431, 8.001804) end of major axis (5.74144, 8.319082) minor radius 0.000037 (5.74144, 8.319082) -> (4.223538, 8.175354) ccw
  ellipse E325 centre (2.485719, 7.006259) end of major axis (5.835728, 7.323536) minor radius 0.000037 (5.59446, 7.3007) -> (4.317921, 7.179817) ccw
  line L396 (5.74144, 8.319082) -> (5.769745, 8.020221)
  ellipse E326 centre (0.901689, 23.731415) end of major axis (3.151621, 23.944505) minor radius 0.000025 (3.151621, 23.944505) -> (1.986589, 23.834188) ccw
  line L397 (3.151621, 23.944505) -> (3.429585, 21.98943)
  line L398 (7.168554, -28.470007) -> (6.503033, -26.754752)
  line L399 (9.243274, -28.470165) -> (8.701158, -26.589519)
  line L400 (-9.790726, -28.468717) -> (-9.892659, -26.449481)
  line L401 (-7.720441, -28.468875) -> (-7.617758, -26.517939)
  line L402 (7.124098, -27.807489) -> (6.891004, -26.707333)
  line L403 (9.255151, -27.754033) -> (9.113723, -26.499134)
  line L404 (-9.248404, -27.752626) -> (-9.106785, -26.497748)
  line L405 (-7.117359, -27.806406) -> (-6.884097, -26.706286)
  line L406 (7.727079, -28.470049) -> (7.624693, -26.519098)
  line L407 (9.797365, -28.470207) -> (9.898638, -26.470054)
  line L408 (-9.236636, -28.468759) -> (-8.69199, -26.580417)
  line L409 (-7.161916, -28.468917) -> (-6.496134, -26.753764)
  line L410 (7.403177, -27.059312) -> (7.320517, -26.613701)
  line L411 (9.589081, -27.074049) -> (9.528435, -26.452763)
  line L412 (-9.582231, -27.072591) -> (-9.52149, -26.451314)
  line L413 (-7.396324, -27.058187) -> (-7.313597, -26.612588)
  ellipse E327 centre (-10.418462, -13.218146) end of major axis (-10.491815, -13.042877) minor radius 0.172083 (-10.593269, -13.209968) -> (-10.487356, -13.384791) ccw
  ellipse E328 centre (-10.47712, -13.242695) end of major axis (-10.403768, -13.417965) minor radius 0.172083 (-10.612447, -13.350888) -> (-10.554235, -13.404679) ccw
  ellipse E329 centre (-10.407301, -16.022023) end of major axis (-10.480654, -15.846753) minor radius 0.172083 (-10.519523, -15.870152) -> (-10.539697, -15.889873) ccw
  ellipse E330 centre (-10.668489, -13.241021) end of major axis (-10.677368, -13.430813) minor radius 0.073999 (-10.663785, -13.428281) -> (-10.594189, -13.209925) ccw
  ellipse E331 centre (-10.806494, -13.234565) end of major axis (-10.815373, -13.424357) minor radius 0.073999 (-10.80179, -13.421824) -> (-10.732194, -13.203469) ccw
  ellipse E332 centre (-10.736675, -16.013892) end of major axis (-10.727796, -15.8241) minor radius 0.073999 (-10.662375, -15.982796) -> (-10.741379, -15.826633) ccw
  ellipse E333 centre (-10.348643, -15.997473) end of major axis (-10.421996, -15.822204) minor radius 0.172083 (-10.452798, -15.839415) -> (-10.52345, -15.989296) ccw
  ellipse E334 centre (-10.59867, -16.020348) end of major axis (-10.589791, -15.830556) minor radius 0.073999 (-10.52437, -15.989253) -> (-10.589791, -15.830556) ccw
  line L414 (-10.589791, -15.830556) -> (-10.727796, -15.8241)
  line L415 (-10.314505, -13.437342) -> (-10.405553, -13.433083)
  line L416 (-10.33173, -13.409243) -> (-10.212791, -13.414807)
  line L417 (-9.727604, -15.679741) -> (-9.738521, -15.245165)
  line L418 (-9.773665, -13.846147) -> (-9.778606, -13.649452)
  line L419 (-11.039481, -13.521301) -> (-10.80179, -13.421824)
  line L420 (-10.663785, -13.428281) -> (-10.794448, -13.482965)
  line L421 (-10.741379, -15.826633) -> (-10.841965, -15.868729)
  line L422 (-11.062838, -15.771939) -> (-11.113841, -13.74165)
  line L423 (-10.145734, -15.819926) -> (-10.227168, -15.816117)
  line L424 (-10.975835, -13.748106) -> (-10.924833, -15.778395)
  line L425 (-9.719948, -13.624903) -> (-9.714052, -13.859613)
  line L426 (-9.688223, -14.887804) -> (-9.668946, -15.655192)
  ellipse E335 centre (-10.511782, -11.862887) end of major axis (-10.585135, -11.687618) minor radius 0.172083 (-10.585135, -11.687618) -> (-10.644178, -11.730737) ccw
  ellipse E336 centre (-10.372639, -17.401831) end of major axis (-10.299287, -17.5771) minor radius 0.172083 (-10.507966, -17.510023) -> (-10.496228, -17.524769) ccw
  ellipse E337 centre (-10.313981, -17.377281) end of major axis (-10.387334, -17.202012) minor radius 0.172083 (-10.488788, -17.369104) -> (-10.42929, -17.509134) ccw
  ellipse E338 centre (-10.453124, -11.838338) end of major axis (-10.526477, -11.663069) minor radius 0.172083 (-10.511672, -11.657733) -> (-10.62793, -11.83016) ccw
  line L427 (-10.585135, -11.687618) -> (-10.526477, -11.663069)
  line L428 (-10.346239, -17.590105) -> (-9.332981, -17.637508)
  line L429 (-10.488788, -17.369104) -> (-10.52345, -15.989296)
  line L430 (-9.921604, -17.582677) -> (-10.272417, -17.566265)
  line L431 (-10.24401, -11.661081) -> (-10.195438, -11.663354)
  line L432 (-10.593269, -13.209968) -> (-10.62793, -11.83016)
  ellipse E339 centre (-9.90241, -15.671563) end of major axis (-9.829058, -15.846833) minor radius 0.172083 (-9.762425, -15.794196) -> (-9.727604, -15.679741) ccw
  ellipse E340 centre (-9.953413, -13.641275) end of major axis (-9.88006, -13.816544) minor radius 0.172083 (-9.778606, -13.649452) -> (-9.786615, -13.597728) ccw
  ellipse E341 centre (-10.988538, -15.740843) end of major axis (-10.997416, -15.930636) minor radius 0.073999 (-11.062838, -15.771939) -> (-11.046698, -15.873738) ccw
  ellipse E342 centre (-11.03954, -13.710554) end of major axis (-11.030661, -13.520762) minor radius 0.073999 (-11.057139, -13.531595) -> (-11.113841, -13.74165) ccw
  ellipse E343 centre (-9.894755, -13.616725) end of major axis (-9.968107, -13.441456) minor radius 0.172083 (-9.719948, -13.624903) -> (-9.747992, -13.526155) ccw